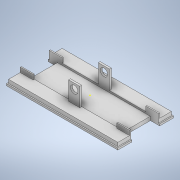
# Autodesk Inventor part: podstawka_pelna
Saved by Autodesk Inventor 2020.3 (Build 243373000, 373)
## iProperties
Created: 2021-01-12
Part Number: podstawka_pelna
Material: Ogólny
Document SubType Name: Modeling
Designer: sitar
Density: 1 g/cm^3
Appearance: Domyślna
Author: sitar
Autodesk Inventor part; units mm, degrees
ref_plane "YZ Plane" through (0, 0, 0) normal (1, 0, 0) x (0, 1, 0)
ref_plane "XZ Plane" through (0, 0, 0) normal (0, 1, 0) x (-1, 0, 0)
ref_plane "XY Plane" through (0, 0, 0) normal (0, 0, 1) x (1, 0, 0)
sketch "Szkic1" plane through (0, 0, 0) normal (0, 1, 0) x (-1, 0, 0)
  point P0 (0, 0)
sketch "Szkic2" plane through (0, 0, 0) normal (0, 1, 0) x (-1, 0, 0)
  line L0 (60, -30) -> (-60, -30)
  line L1 (-60, -30) -> (-60, 30)
  line L2 (-60, 30) -> (60, 30)
  line L3 (60, 30) -> (60, -30)
  line L4 (60, -30) -> (-60, 30) construction
  line L5 (-60, -30) -> (60, 30) construction
  point P0 (0, 0)
  dimension "d0" = 120
  dimension "d1" = 60
  constraints: 12 end point, 2 midpoint, 2 parallel, 1 horizontal, 1 perpendicular
  measures "d0" distance of L1.end L2.end
  measures "d1" distance of L0.end L1.end
extrude "Wyciągnięcie proste1" add sketch "Szkic2" along normal blind 10
sketch "Szkic3" plane through (0, 10, 0) normal (0, 1, 0) x (1, 0, 0)
  line L0 (0, 0) -> (50, 0)
  line L1 (60, -30) -> (60, 30) projected
  line L2 (50, 0) -> (60, 0)
  line L3 (60, 0) -> (60, 15)
  line L4 (60, 15) -> (50, 15)
  line L5 (50, 15) -> (50, 0)
  dimension "d4" = 50
  dimension "d5" = 15
  constraints: 10 end point, 2 horizontal, 2 parallel, 1 perpendicular, 1 point on line
  measures "d4" distance of L0.start L0.end
  measures "d5" distance of L3.end L2.end
extrude "Wyciągnięcie proste2" cut sketch "Szkic3" against normal blind 10
mirror "Odbij1" about plane through (0, 0, 0) normal (0, 0, 1) of "Wyciągnięcie proste2"
mirror "Odbij2" about plane through (0, 0, 0) normal (1, 0, 0) of "Wyciągnięcie proste2"
mirror "Odbij3" about plane through (0, 0, 0) normal (0, 0, 1) of "Wyciągnięcie proste2", "Odbij2"
sketch "Szkic4" plane through (0, 10, 0) normal (0, 1, 0) x (1, 0, 0)
  line L0 (-50, 15) -> (50, 15)
  line L1 (50, 15) -> (50, -15)
  line L2 (50, -15) -> (-50, -15)
  line L3 (-50, -15) -> (-50, 15)
  line L4 (-50, 15) -> (50, -15) construction
  line L5 (50, 15) -> (-50, -15) construction
  point P0 (0, 0)
  constraints: 12 end point, 2 midpoint, 2 parallel, 1 horizontal, 1 perpendicular
extrude "Wyciągnięcie proste3" cut sketch "Szkic4" against normal blind 2
sketch "Szkic5" plane through (0, 10, 0) normal (0, 1, 0) x (1, 0, 0)
  line L0 (0, 0) -> (0, -16)
  line L1 (50, -15) -> (-50, -15) projected
  line L2 (0, 0) -> (16, 0) construction
  line L3 (-6, -15) -> (6, -15)
  line L4 (6, -15) -> (6, -17)
  line L5 (6, -17) -> (-6, -17)
  line L6 (-6, -17) -> (-6, -15)
  line L7 (-6, -15) -> (6, -17) construction
  line L8 (6, -15) -> (-6, -17) construction
  dimension "d10" = 16
  dimension "d11" = 90
  dimension "d12" = 12
  dimension "d13" = 2
  constraints: 16 end point, 3 perpendicular, 2 horizontal, 2 midpoint, 2 parallel
  measures "d10" distance of L0.start L0.end
  measures "d11" angle of L0 L2
  measures "d12" distance of L4.end L5.end
  measures "d13" distance of L3.end L4.end
extrude "Wyciągnięcie proste4" add sketch "Szkic5" along normal blind 20
sketch "Szkic6" plane through (-6, 10, 17) normal (0, 0, 1) x (1, 0, 0)
  point P0 (6, -10)
sketch "Szkic7" plane through (-6, 10, 17) normal (0, 0, 1) x (1, 0, 0)
  line L0 (12, 20) -> (0, 20) projected
  line L1 (6, 20) -> (6, 14)
  line L2 (6, 20) -> (12, 20) construction
  circle A0 centre (6, 14) radius 4
  point P0 (6, -10)
  dimension "d16" = 6
  dimension "d17" = 90
  dimension "d18" = 8
  constraints: 4 end point, 1 centre point, 1 coincident, 1 horizontal, 1 midpoint, 1 perpendicular, 1 vertical
  measures "d16" distance of L1.start L1.end
  measures "d17" angle of L1 L2
  measures "d18" diameter of A0
extrude "Wyciągnięcie proste5" cut sketch "Szkic7" against normal through all
sketch "Szkic8" plane through (0, 10, 0) normal (0, 1, 0) x (1, 0, 0)
  point P0 (0, 0)
mirror "Odbij4" about plane through (0, 0, 0) normal (0, 0, 1) of "Wyciągnięcie proste4", "Wyciągnięcie proste5"
sketch "Szkic9" plane through (0, 10, 0) normal (0, 1, 0) x (1, 0, 0)
  line L0 (6, 15) -> (60, 15) projected
  line L1 (60, 15) -> (45, 15)
  line L2 (45, 15) -> (45, 16.2)
  line L3 (45, 16.2) -> (60, 16.2)
  line L4 (60, 16.2) -> (60, 15)
  point P0 (0, 0)
  dimension "d21" = 15
  dimension "d22" = 1.2
  constraints: 8 end point, 2 parallel, 1 horizontal, 1 perpendicular
  measures "d21" distance of L2.end L3.end
  measures "d22" distance of L1.end L2.end
extrude "Wyciągnięcie proste6" add sketch "Szkic9" along normal blind 5
mirror "Odbij5" about plane through (0, 0, 0) normal (1, 0, 0) of "Wyciągnięcie proste6"
mirror "Odbij6" about plane through (0, 0, 0) normal (0, 0, 1) of "Wyciągnięcie proste6"
sketch "Szkic10" plane through (0, 10, 0) normal (0, 1, 0) x (1, 0, 0)
  line L0 (60, 30) -> (-60, 30) projected
  line L1 (60, 15) -> (60, 30) projected
  line L2 (-60, 30) -> (60, 30)
  line L3 (60, 30) -> (60, 28.8)
  line L4 (60, 28.8) -> (-60, 28.8)
  line L5 (-60, 28.8) -> (-60, 30)
  point P0 (0, 0)
  dimension "d25" = 1.2
  constraints: 8 end point, 2 parallel, 1 horizontal, 1 perpendicular, 1 point on line
  measures "d25" distance of L2.end L3.end
extrude "Wyciągnięcie proste7" cut sketch "Szkic10" against normal blind 4
mirror "Odbij7" about plane through (0, 0, 0) normal (0, 0, 1) of "Wyciągnięcie proste7"
sketch "Szkic11" plane through (0, 10, 0) normal (0, 1, 0) x (1, 0, 0)
  point P0 (0, 0)
sketch "Szkic12" plane through (0, 15, 0) normal (0, 1, 0) x (1, 0, 0)
  line L0 (60, 28.8) -> (-60, 28.8) projected
  line L1 (-60, -28.8) -> (60, -28.8) projected
  line L2 (60, 28.8) -> (58.8, 28.8)
  line L3 (58.8, 28.8) -> (58.8, -28.8)
  line L4 (58.8, -28.8) -> (60, -28.8)
  line L5 (60, -28.8) -> (60, 28.8)
  point P0 (0, 0)
  dimension "d28" = 1.2
  constraints: 8 end point, 2 parallel, 1 horizontal, 1 perpendicular, 1 point on line
  measures "d28" distance of L4.end L3.end
extrude "Wyciągnięcie proste8" cut sketch "Szkic12" against normal up to surface (9 mm away)
mirror "Odbij8" about plane through (0, 0, 0) normal (1, 0, 0) of "Wyciągnięcie proste8"
sketch "Szkic13" plane through (0, 0, 0) normal (0, -1, 0) x (1, 0, 0)
  line L0 (60, -30) -> (-60, -30) projected
  line L1 (60, -30) -> (-60, -30)
  line L2 (-60, -30) -> (-60, 30)
  line L3 (-60, 30) -> (60, 30)
  line L4 (60, 30) -> (60, -30)
  point P0 (0, 0)
  constraints: 8 end point, 2 parallel, 1 horizontal, 1 perpendicular
extrude "Wyciągnięcie proste9" cut sketch "Szkic13" against normal blind 4
mirror "Odbij9" about plane through (0, 0, 0) normal (0, 0, 1) of "Wyciągnięcie proste6", "Odbij5"
sketch "Szkic14" plane through (-60, 10, 15) normal (-1, 0, 0) x (0, 0, 1)
  line L0 (1.2, 0) -> (1.2, 5) projected
  line L1 (0, 0) -> (0, 20) projected
  line L2 (1.2, 5) -> (0, 5)
  line L3 (0, 5) -> (0, 0)
  line L4 (0, 0) -> (1.2, 0)
  line L5 (1.2, 0) -> (1.2, 5)
  point P0 (-15, -10)
  constraints: 8 end point, 2 parallel, 1 horizontal, 1 perpendicular
extrude "Wyciągnięcie proste10" cut sketch "Szkic14" against normal up to surface (1.2 mm away)
sketch "Szkic15" plane through (58.8, 10, 15) normal (0, -1, 0) x (1, 0, 0)
  line L0 (1.2, 1.2) -> (-13.8, 1.2) projected
  line L1 (0, 0) -> (1.2, 0)
  line L2 (1.2, 0) -> (1.2, 1.2)
  line L3 (1.2, 1.2) -> (0, 1.2)
  line L4 (0, 1.2) -> (0, 0)
  point P0 (-58.8, -15)
  constraints: 8 end point, 2 parallel, 1 horizontal, 1 perpendicular
extrude "Wyciągnięcie proste11" cut sketch "Szkic15" against normal blind 10
